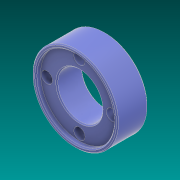
# Autodesk Inventor part: spacer nema23
Saved by Autodesk Inventor 2020.2 (Build 242310000, 310)
## iProperties
Created: 2020-05-18
Part Number: spacer nema23
Material: PC/ABS Plastic
Document SubType Name: Modeling
Designer: Svend
Density: 0.357273 g/cm^3
Appearance: Smooth - White
Author: Svend
Autodesk Inventor part; units mm, degrees
ref_plane "YZ Plane" through (0, 0, 0) normal (1, 0, 0) x (0, 1, 0)
ref_plane "XZ Plane" through (0, 0, 0) normal (0, 1, 0) x (-1, 0, 0)
ref_plane "XY Plane" through (0, 0, 0) normal (0, 0, 1) x (1, 0, 0)
sketch "Sketch1" plane through (0, 0, 0) normal (0, 0, 1) x (1, 0, 0)
  circle A0 centre (0, 0) radius 21
  circle A1 centre (16, 0) radius 2.75
  circle A2 centre (0, 16) radius 2.75
  circle A3 centre (-16, 0) radius 2.75
  circle A4 centre (0, -16) radius 2.75
  circle A5 centre (0, 0) radius 11.1
  dimension "d0" = 42
  dimension "d1" = 5.5
  dimension "d2" = 16
  dimension "d5" = 360
  dimension "d7" = 22.2
  constraints: 6 centre point, 2 coincident, 1 horizontal alignment, 9 other
  measures "d0" diameter of A0
  measures "d1" diameter of A1
  measures "d2" distance of point (0, 0) A1.centre
  measures "d7" diameter of A5
extrude "Extrusion1" add sketch "Sketch1" along normal blind 15
sketch "Sketch2" plane through (0, 0, 15) normal (0, 0, 1) x (1, 0, 0)
  circle A0 centre (0, 0) radius 19.1
  dimension "d10" = 38.2
  constraints: 1 centre point, 1 coincident
  measures "d10" diameter of A0
extrude "Extrusion2" cut sketch "Sketch2" against normal blind 2.3
chamfer "Chamfer1" distance 0.5 angle 45 9 edges at (-21, 0, 0) (-21, 0, 15) (-11.1, 0, 0) (-2.75, -16, 0) (-2.75, 16, 0) (13.25, 0, 0) (-18.75, 0, 0) (-11.1, 0, 12.7) (-19.1, 0, 15)
body "Solid1"
